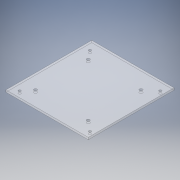
# Autodesk Inventor part: Acrylic_Vesa
Saved by Autodesk Inventor 2019 (Build 230136000, 136)
## iProperties
Created: 2019-05-23
Part Number: Acrylic_Vesa
Material: PET Plastic
Document SubType Name: Modeling
Designer: Jorian Bruslind
Density: 1.541 g/cm^3
Appearance: Polycarbonate - Clear
Author: Jorian Bruslind
Autodesk Inventor part; units mm, degrees
ref_plane "YZ Plane" through (0, 0, 0) normal (1, 0, 0) x (0, 1, 0)
ref_plane "XZ Plane" through (0, 0, 0) normal (0, 1, 0) x (-1, 0, 0)
ref_plane "XY Plane" through (0, 0, 0) normal (0, 0, 1) x (1, 0, 0)
sketch "Sketch1" plane through (0, 0, 0) normal (0, 1, 0) x (-1, 0, 0)
  line L0 (0, 0) -> (117, 0)
  line L1 (117, 0) -> (117, -122)
  line L2 (117, -122) -> (0, -122)
  line L3 (0, -122) -> (0, 0)
  dimension "d0" = 117
  dimension "d1" = 122
  constraints: 8 end point, 2 parallel, 1 horizontal, 1 perpendicular
  measures "d0" distance of L1.end L2.end
  measures "d1" distance of L0.end L1.end
extrude "Extrusion1" add sketch "Sketch1" along normal blind 3
sketch "Sketch2" plane through (0, 3, 0) normal (0, 1, 0) x (1, 0, 0)
  line L0 (-117, 0) -> (0, 0) projected
  line L1 (-117, 0) -> (-117, 21)
  line L2 (-117, 122) -> (-117, 0) projected
  line L3 (-117, 21) -> (-96, 21)
  circle A0 centre (-96, 21) radius 2.1
  circle A1 centre (-96, 96) radius 2.1
  circle A2 centre (-21, 21) radius 2.1
  circle A3 centre (-21, 96) radius 2.1
  line L4 (-117, 0) -> (-117, 8.5)
  line L5 (-117, 8.5) -> (-106, 8.5)
  circle A4 centre (-106, 8.5) radius 1.75
  circle A5 centre (-106, 108.5) radius 1.75
  circle A6 centre (-6, 8.5) radius 1.75
  circle A7 centre (-6, 108.5) radius 1.75
  dimension "d4" = 21
  dimension "d5" = 21
  dimension "d6" = 4.2
  dimension "d9" = 75
  dimension "d12" = 75
  dimension "d15" = 8.5
  dimension "d16" = 11
  dimension "d17" = 3.5
  dimension "d20" = 100
  dimension "d23" = 100
  constraints: 8 centre point, 8 end point, 2 coincident, 2 horizontal, 2 perpendicular, 2 point on line, 2 vertical, 12 other
  measures "d4" distance of L0.start L1.end
  measures "d5" distance of L1.end L3.end
  measures "d6" diameter of A0
  measures "d9" distance of A0.centre A1.centre
  measures "d12" distance of A0.centre A2.centre
  measures "d15" distance of L0.start L4.end
  measures "d16" distance of L4.end L5.end
  measures "d17" diameter of A4
  measures "d20" distance of A4.centre A5.centre
  measures "d23" distance of A4.centre A6.centre
extrude "Extrusion2" cut sketch "Sketch2" against normal blind 3
body "Solid1"
